Autodesk Fusion 360 part; units mm, degrees
(part 5 of 5)
  constraint perpendicular L8 L9
  constraint parallel L8 L10
  constraint parallel L9 L11
  constraint coincident P0 L0.end
  constraint coincident P1 L1.end
  constraint coincident P3 L0.start
  constraint coincident P9 L15.start
  constraint coincident P10 L15.end
  constraint coincident P11 L16.end
  constraint coincident P8 L17.start
  constraint coincident P15 L18.start
  constraint coincident P12 L19.start
  constraint coincident P13 L20.start
  constraint coincident P14 L20.end
  constraint midpoint L12 A0.centre
  constraint midpoint L13 A1.centre
  constraint midpoint L14 A2.centre
  constraint coincident P2 L2.end
  constraint midpoint L23 A3.centre
  constraint equal A0 A1
  constraint equal A1 A3
  constraint equal A2 A3
  constraint horizontal L64
  constraint perpendicular L57 L64
  constraint parallel L57 L62
  constraint coincident P28 P16
  constraint coincident P17 L55.start
  constraint coincident P18 L54.start
  constraint coincident P24 L59.end
  constraint coincident P29 L58.end
  constraint coincident P20 L70.start
  constraint coincident P30 L63.end
  constraint coincident P22 L56.end
  constraint coincident P33 L56.start
  constraint coincident P31 L58.start
  constraint coincident P32 L65.start
  constraint coincident P23 L65.end
  constraint midpoint A7.centre L73
  constraint midpoint A4.centre L54
  constraint midpoint A6.centre L68
  constraint coincident P19 L59.start
  constraint midpoint A5.centre L67
  constraint equal A4 A7
  constraint equal A4 A5
  constraint equal A5 A6
  constraint horizontal L123
  constraint perpendicular L123 L131
  constraint parallel L130 L131
  constraint coincident P46 P40
  constraint coincident P39 L126.start
  constraint coincident P38 L120.start
  constraint coincident P37 L118.end
  constraint coincident P47 L119.start
  constraint coincident P42 L119.end
  constraint coincident P48 L128.end
  constraint coincident P35 L117.end
  constraint coincident P44 L117.start
  constraint coincident P52 L129.start
  constraint coincident P50 L133.start
  constraint coincident P36 L125.start
  constraint midpoint A11.centre L132
  constraint midpoint A10.centre L122
  constraint midpoint A9.centre L121
  constraint coincident P41 L118.start
  constraint midpoint A8.centre L127
  constraint equal A10 A11
  constraint equal A8 A10
  constraint equal A8 A9
  measures "d633" distance of P2 L11
  measures "d634" distance of P3 L9
  measures "d635" distance of P0 L10
  measures "d636" distance of P3 L8
  measures "d637" diameter of A0
  measures "d664" distance of P19 L62
  measures "d665" distance of P24 L57
  measures "d666" distance of P17 L69
  measures "d667" distance of P24 L64
  measures "d668" diameter of A7
  measures "d670" distance of P41 L130
  measures "d671" distance of P37 L131
  measures "d672" distance of P39 L124
  measures "d673" distance of P37 L123
  measures "d674" diameter of A11
extrude "Extrude4''''" add sketch "Sketch2 (5)" along normal blind 3.6 separate body contours L0 L3 L22 | L0 L1 L15 | L2 L3 L21 | L1 L2 L17 | L8 L9 L10 L11 | L24 S0 S1 S2 S3 S4 S5 S6 L25 S7 S8 S9 S10 S11 S12 S13 L26 S14 S15 S16 S17 S18 S19 S20 S21 S22 S23 S24 S25 S26 | L27 L28 L29 L30 | L31 S27 S28 S29 S30 S31 S32 S33 S34 S35 S36 S37 S38 S39 S40 S41 S42 S43 S44 | S45 S46 S47 S48 S49 S50 S51 S52 S53 | L32 L33 L34 S54 S55 S56 S57 S58 S59 S60 L35 L36 L37 S61 S62 S63 S64 S65 L38 L39 L40 S66 S67 S68 S69 S70 L41 L42 | L43 L44 L45 S71 S72 S73 S74 S75 S76 S77 L46 L47 L48 S78 S79 S80 S81 S82 L49 L50 L51 S83 S84 S85 S86 S87 L52 L53 picked at (11.9917, 14.9333) picked at (11.9917, -11.1667) picked at (-11.9917, 14.9333) picked at (-11.9917, -11.1667) picked at (16.2215, -1.3333) picked at (4.9489, -15.6243) picked at (3.366, -14.1398) picked at (2.568, -15.6926) picked at (1.6677, -15.419) picked at (0.132, -15.1003) picked at (-3.3591, -15.1003) makes body 21 in component "display trial"
extrude "Extrude5''''" cut sketch "Sketch1 (7)" along normal blind 2.5 from surface at -4 contours A0 | A1 | A2 | A3 picked at (-16.5962, -15.4559) picked at (16.6171, -15.5472) picked at (16.0634, 19.1784) picked at (-16.4833, 19.2742) bodies 20 in component "display trial"
extrude "Extrude53" cut sketch "Display cutout (2)" against normal blind 2.5 contours A0 | A1 | A2 | A3 picked at (-46.5866, -131.8202) picked at (-13.9366, -131.8202) picked at (-46.0119, -97.0946) picked at (-13.6923, -97.7089) bodies 5 in component "GM67 + printer"
extrude "Extrude54" cut sketch "SCanner support" against normal up to surface (4 mm away) contours A8 | A9 picked at (14.888, -97.705) picked at (48.012, -96.756) bodies 5 in component "GM67 + printer"
extrude "Extrude55" add sketch "Display cutout (2)" along normal up to surface (1.5 mm away) from surface at -4 contours L14 L22 L23 L24 L25 L33 | L15 L22 L23 L24 L25 L34 picked at (-16.675, -118.5474) picked at (-42.825, -118.5474) bodies 5 in component "GM67 + printer"
extrude "Extrude6'''" add sketch "Sketch2 (5)" along normal blind 3.4 separate body contours L55 L61 L71 | L55 L60 L63 | L59 L61 L66 | L59 L60 L72 | L57 L62 L64 L69 | L74 S88 S89 S90 S91 S92 S93 S94 L75 S95 S96 S97 S98 S99 S100 S101 L76 S102 S103 S104 S105 S106 S107 S108 S109 S110 S111 S112 S113 S114 | L77 L78 L79 L80 | L81 L82 L83 L84 L85 L86 L87 L88 L89 L90 L91 | L92 L93 L94 | L95 L96 L97 S115 S116 S117 S118 S119 S120 S121 L98 L99 L100 S122 S123 S124 S125 S126 L101 L102 L103 S127 S128 S129 S130 S131 L104 L105 | L106 L107 L108 S132 S133 S134 S135 S136 S137 S138 L109 L110 L111 S139 S140 S141 S142 S143 L112 L113 L114 S144 S145 S146 S147 S148 L115 L116 picked at (-59.0083, -11.1667) picked at (-82.9917, -11.1667) picked at (-59.0083, 14.9333) picked at (-82.9917, 14.9333) picked at (-54.7785, -1.3333) picked at (-66.0511, -15.6243) picked at (-67.634, -14.1398) picked at (-69.7384, -16.1548) picked at (-69.1797, -15.5068) picked at (-70.868, -15.1003) picked at (-74.3591, -15.1003) makes body 22 in component "display trial"
extrude "Extrude7''" add sketch "Sketch2 (5)" along normal blind 3.2 separate body contours L118 L120 L125 | L120 L126 L134 | L118 L135 L136 | L119 L126 L136 | L123 L124 L130 L131 | L137 S149 S150 S151 S152 S153 S154 S155 L138 S156 S157 S158 S159 S160 S161 S162 L139 S163 S164 S165 S166 S167 S168 S169 S170 S171 S172 S173 S174 S175 | L140 L141 L142 L143 | L144 L145 S176 S177 S178 S179 S180 S181 S182 S183 S184 L146 S185 S186 S187 S188 S189 S190 S191 S192 S193 L147 | L148 L149 L150 S194 S195 S196 S197 S198 S199 S200 L151 L152 L153 S201 S202 S203 S204 S205 L154 L155 L156 S206 S207 S208 S209 S210 L157 L158 | L159 L160 L161 S211 S212 S213 S214 S215 S216 S217 L162 L163 L164 S218 S219 S220 S221 S222 L165 L166 L167 S223 S224 S225 S226 S227 L168 L169 picked at (-137.9917, 14.9333) picked at (-137.9917, -11.1667) picked at (-114.0083, 14.9333) picked at (-114.0083, -11.1667) picked at (-109.7785, -1.3333) picked at (-121.0511, -15.6243) picked at (-122.634, -14.1398) picked at (-124.0965, -14.118) picked at (-125.868, -15.1003) picked at (-129.3591, -15.1003) makes body 23 in component "display trial"
extrude "Extrude8'''" cut sketch "Sketch2 (5)" against normal blind 1.5 from surface at 3.6 contours L24 S0 S1 S2 S3 S4 S5 S6 L25 S8 S9 S10 S11 S12 S13 L26 S14 S15 S16 S17 S18 S19 S20 S21 S22 S23 S24 S25 S26 | L27 L28 L29 L30 | L31 S27 S28 S29 S30 S31 S32 S33 S34 S35 S36 S37 S38 S39 S40 S41 S42 S43 S44 | L32 L33 L34 S54 S55 S56 S57 S58 S59 S60 L35 L36 L37 S61 S62 S63 S64 S65 L38 L39 L40 S66 S67 S68 S69 S70 L41 L42 | L43 L44 L45 S71 S72 S73 S74 S75 S76 S77 L46 L47 L48 S78 S79 S80 S81 S82 L49 L50 L51 S83 S84 S85 S86 S87 L52 L53 picked at (4.9451, -15.6266) picked at (3.366, -14.1398) picked at (2.568, -15.6926) picked at (0.132, -15.1003) picked at (-3.3591, -15.1003) bodies 21 in component "display trial"
extrude "Extrude9" cut sketch "Sketch2 (5)" against normal blind 1.5 from surface at 3.4 contours L74 S88 S89 S90 S91 S92 S93 S94 L75 S96 S97 S98 S99 S100 S101 L76 S102 S103 S104 S105 S106 S107 S108 S109 S110 S111 S112 S113 S114 | L77 L78 L79 L80 | L81 L82 L83 L84 L85 L86 L87 L88 L89 L90 L91 | L95 L96 L97 S115 S116 S117 S118 S119 S120 S121 L98 L99 L100 S122 S123 S124 S125 S126 L101 L102 L103 S127 S128 S129 S130 S131 L104 L105 | L106 L107 L108 S132 S133 S134 S135 S136 S137 S138 L109 L110 L111 S139 S140 S141 S142 S143 L112 L113 L114 S144 S145 S146 S147 S148 L115 L116 picked at (-66.0549, -15.6266) picked at (-67.634, -14.1398) picked at (-69.7384, -16.1548) picked at (-70.868, -15.1003) picked at (-74.3591, -15.1003) bodies 22 in component "display trial"
extrude "Extrude10" cut sketch "Sketch2 (5)" against normal blind 1.5 from surface at 3.2 contours L137 S149 S150 S151 S152 S153 S154 S155 L138 S157 S158 S159 S160 S161 S162 L139 S163 S164 S165 S166 S167 S168 S169 S170 S171 S172 S173 S174 S175 | L140 L141 L142 L143 | L144 L145 S176 S177 S178 S179 S180 S181 S182 S183 S184 L146 S185 S186 S187 S188 S189 S190 S191 S192 S193 L147 | L148 L149 L150 S194 S195 S196 S197 S198 S199 S200 L151 L152 L153 S201 S202 S203 S204 S205 L154 L155 L156 S206 S207 S208 S209 S210 L157 L158 | L159 L160 L161 S211 S212 S213 S214 S215 S216 S217 L162 L163 L164 S218 S219 S220 S221 S222 L165 L166 L167 S223 S224 S225 S226 S227 L168 L169 picked at (-121.0549, -15.6266) picked at (-122.634, -14.1398) picked at (-124.0965, -14.118) picked at (-125.868, -15.1003) picked at (-129.3591, -15.1003) bodies 23 in component "display trial"
sketch "Sketch1 (8)" plane through (0, 0, 0) normal (0, 1, 0) x (1, 0, 0) in component "Bottom LID - Printer"
  line L0 (0, -115) -> (4, -115)
  arc A0 (19, -100) -> (4, -115) centre (19, -115) ccw
  line L1 (19, -100) -> (43.5, -100)
  arc A1 (43.5, -100) -> (53.5, -90) centre (43.5, -90) ccw
  line L2 (53.5, -90) -> (53.5, -10)
  arc A2 (53.5, -10) -> (43.5, 0) centre (43.5, -10) ccw
  line L3 (43.5, 0) -> (0, 0)
  line L4 (0, 0) -> (0, -115)
  line L5 (49.5, -10) -> (49.5, -90)
  arc A3 (43.5, -96) -> (49.5, -90) centre (43.5, -90) ccw
  line L6 (43.5, -96) -> (4, -96)
  line L7 (4, -96) -> (4, -4)
  line L8 (4, -4) -> (43.5, -4)
  arc A4 (49.5, -10) -> (43.5, -4) centre (43.5, -10) ccw
  line L9 (12, -4) -> (4, -4)
  line L10 (4, -4) -> (4, -12)
  arc A5 (4, -12) -> (12, -4) centre (4, -4) ccw
  line L11 (4, -88) -> (4, -96)
  line L12 (4, -96) -> (12, -96)
  arc A6 (12, -96) -> (4, -88) centre (4, -96) ccw
  arc A7 (45.5, -10) -> (43.5, -8) centre (43.5, -10) ccw
  arc A8 (43.5, -92) -> (45.5, -90) centre (43.5, -90) ccw
  line L13 (45.5, -10) -> (45.5, -90)
  arc A9 (8, -15.3137) -> (15.3137, -8) centre (4, -4) ccw
  arc A10 (15.3137, -92) -> (8, -84.6863) centre (4, -96) ccw
  line L14 (15.3137, -8) -> (43.5, -8)
  line L15 (8, -84.6863) -> (8, -15.3137)
  line L16 (43.5, -92) -> (15.3137, -92)
  circle A11 centre (6.8284, -6.8284) radius 1.75
  circle A12 centre (6.8284, -6.8284) radius 2.8
  circle A13 centre (6.8284, -93.1716) radius 1.75
  circle A14 centre (6.8284, -93.1716) radius 2.8
  line L17 (15.3137, -92) -> (15.3137, -96)
  line L18 (15.3137, -8) -> (15.3137, -4)
  line L19 (40.3137, -96) -> (40.3137, -92)
  line L20 (40.3137, -8) -> (40.3137, -4)
  point P0 (6.8284, -6.8284)
  point P1 (6.8284, -93.1716)
  dimension "d698" = 3.5
  dimension "d699" = 5.6
  dimension "d707" = 25
  constraint concentric A5 A9
  constraint concentric A4 A7
  constraint concentric A3 A8
  constraint tangent A8 L16
  constraint tangent A7 L13
  constraint tangent A8 L13
  constraint coincident P0 A11.centre
  constraint concentric A11 A12
  constraint coincident P1 A13.centre
  constraint equal A12 A14
  constraint equal A11 A13
  constraint coincident L6 L17.end
  constraint perpendicular L6 L17
  constraint coincident L8 L18.end
  constraint perpendicular L8 L18
  constraint coincident L6 L19.start
  constraint coincident L16 L19.end
  constraint perpendicular L16 L19
  constraint coincident L14 L20.start
  constraint coincident L8 L20.end
  constraint perpendicular L8 L20
  constraint collinear L19 L20
  measures "d698" diameter of A11
  measures "d699" diameter of A12
  measures "d707" distance of L17 L19.end
extrude "Extrude1''''''''''" add sketch "Sketch1 (8)" against normal blind 8 separate body contours L5 A3 L6 L8 A4 A7 A8 L13 L14 L16 L19 L20 | L8 L14 L18 L20 | L6 L16 L17 L19 | L6 L7 L8 A5 A6 A9 A10 L15 L17 L18 picked at (48.1667, -63.3333) picked at (31.9804, -6.6667) picked at (31.9804, -94.6667) picked at (5.3333, -61.5621) makes body 24 in component "Bottom LID - Printer"
extrude "Extrude3'''''''" add sketch "Sketch1 (8)" along normal blind 4 contours L0 A0 L1 A1 L2 A2 L3 L4 | L5 A3 L6 L8 A4 A7 A8 L13 L14 L16 L19 L20 | L8 L14 L18 L20 | L6 L16 L17 L19 | L6 L7 L8 A5 A6 A9 A10 L15 L17 L18 | A7 A8 L13 A9 A10 L14 L15 L16 | L7 L8 L9 L10 A5 | L6 L7 L11 L12 A6 | A12 | A14 picked at (8.9635, -98.1271) picked at (48.1667, -63.3333) picked at (31.9804, -6.6667) picked at (31.9804, -94.6667) picked at (5.3333, -61.5621) picked at (33.5434, -61.8009) picked at (11.0202, -4.7965) picked at (11.0202, -95.2035) picked at (9.268, -6.9675) picked at (9.268, -93.3107) bodies 24 in component "Bottom LID - Printer"
extrude "Extrude5'''''" add sketch "Sketch1 (8)" against normal blind 2.5 contours L7 L8 L9 L10 A5 | L6 L7 L11 L12 A6 | A12 | A14 picked at (11.0202, -4.7965) picked at (11.0202, -95.2035) picked at (9.268, -6.9675) picked at (9.268, -93.3107) bodies 24 in component "Bottom LID - Printer"
extrude "Extrude6''''" cut sketch "Sketch1 (8)" against normal blind 3 from surface at 4 contours A12 | A14 picked at (9.268, -6.9675) picked at (9.268, -93.3107) bodies 24 in component "Bottom LID - Printer"
extrude "Extrude7'''" add sketch "Sketch1 (8)" against normal blind 5 from surface at -8 contours L8 L14 L18 L20 | L6 L16 L17 L19 picked at (31.9804, -6.6667) picked at (31.9804, -94.6667) bodies 24 in component "Bottom LID - Printer"
fillet "Fillet2'" radius 2 8 edges at (15.3137, -8, 6) (15.3137, -13, 6) (40.3137, -13, 6) (40.3137, -8, 6) (40.3137, -8, 94) (40.3137, -13, 94) (15.3137, -13, 94) (15.3137, -8, 94) on bodies 24 in component "Bottom LID - Printer"
sketch "Sketch1 (9)" plane through (0, 0, 0) normal (0, 1, 0) x (1, 0, 0) in component "Top lid"
  line L0 (0, 0) -> (183.0748, 0)
  line L1 (53.5, -96) -> (53.5, -4)
  line L2 (196.0652, -7.5) -> (240.6025, -84.641)
  line L3 (192.6011, -9.5) -> (237.1384, -86.641)
  line L4 (4, -4) -> (183.0748, -4)
  arc A0 (109.3397, -4) -> (125.3397, -4) centre (117.3397, -4) ccw
  arc A1 (53.5, -12) -> (61.5, -4) centre (53.5, -4) ccw
  arc A2 (61.5, -96) -> (53.5, -88) centre (53.5, -96) ccw
  line L5 (125.3397, -96) -> (19, -96)
  line L6 (125.3397, -100) -> (19, -100)
  arc A3 (141.7942, -105.5) -> (125.3397, -96) centre (125.3397, -115) ccw
  arc A4 (138.3301, -107.5) -> (125.3397, -100) centre (125.3397, -115) ccw
  line L7 (154, -134.641) -> (138.3301, -107.5)
  line L8 (157.4641, -132.641) -> (141.7942, -105.5)
  line L9 (179.9994, -4) -> (179.9994, -6.8969)
  line L10 (181.9766, -9.7171) -> (186.9578, -11.5237)
  arc A5 (179.9994, -6.8969) -> (181.9766, -9.7171) centre (182.9994, -6.8969) ccw
  line L11 (192.6011, -9.5) -> (189.4806, -11.3016)
  arc A6 (196.0652, -7.5) -> (183.0748, 0) centre (183.0748, -15) ccw
  arc A7 (186.9578, -11.5237) -> (189.4806, -11.3016) centre (187.9806, -8.7035) ccw
  arc A8 (154, -134.641) -> (174.4904, -140.1314) centre (166.9904, -127.141) ccw
  arc A9 (157.4641, -132.641) -> (172.4904, -136.6673) centre (166.9904, -127.141) ccw
  spline S0 degree 2 poles (157.4641, -132.641) (166.9904, -127.141) (172.4904, -136.6673) knots 0 0 0 1.944544 1.944544 1.944544 weights 1 3 1
  line L12 (233.1122, -101.6673) -> (172.4904, -136.6673)
  line L13 (235.1122, -105.1314) -> (174.4904, -140.1314)
  arc A10 (233.1122, -101.6673) -> (237.1384, -86.641) centre (227.6122, -92.141) ccw
  spline S1 degree 2 poles (233.1122, -101.6673) (227.6122, -92.141) (237.1384, -86.641) knots 0 0 0 1.944544 1.944544 1.944544 weights 1 3 1
  arc A11 (235.1122, -105.1314) -> (240.6025, -84.641) centre (227.6122, -92.141) ccw
  line L14 (53.5, -4) -> (53.5, 0)
  line L15 (53.5, -96) -> (53.5, -100)
  circle A12 centre (56.3284, -93.1716) radius 1.75
  circle A13 centre (165.1786, -133.9025) radius 1.75
  circle A14 centre (234.3736, -93.9527) radius 1.75
  arc A15 (125.3397, -96) -> (109.3397, -96) centre (117.3397, -96) ccw
  circle A16 centre (117.3397, -93.1716) radius 1.75
  circle A17 centre (56.3284, -6.8284) radius 1.75
  circle A18 centre (117.3397, -6.8284) radius 1.75
  circle A19 centre (185.872, -7.6542) radius 1.75
  circle A20 centre (56.3284, -6.8284) radius 2.75
  circle A21 centre (117.3397, -6.8284) radius 2.75
  circle A22 centre (185.872, -7.6542) radius 2.75
  circle A23 centre (117.3397, -93.1716) radius 2.75
  circle A24 centre (56.3284, -93.1716) radius 2.75
  circle A25 centre (234.3736, -93.9527) radius 2.75
  circle A26 centre (165.1786, -133.9025) radius 2.75
  arc A27 (43.5, -100) -> (53.5, -90) centre (43.5, -90) ccw
  line L16 (43.5, -100) -> (125.3397, -100)
  arc A28 (53.5, -10) -> (43.5, 0) centre (43.5, -10) ccw
  line L17 (183.0748, 0) -> (43.5, 0)
  arc A29 (192.6011, -9.5) -> (183.0748, -4) centre (183.0748, -15) ccw
  line L18 (158.9576, -127.2278) -> (145.2583, -103.5)
  arc A30 (145.2583, -103.5) -> (128.7396, -92.2527) centre (125.3397, -115) ccw
  arc A31 (64.8137, -92) -> (57.5, -84.6863) centre (53.5, -96) ccw
  arc A32 (57.5, -15.3137) -> (64.8137, -8) centre (53.5, -4) ccw
  arc A33 (106.026, -8) -> (128.6534, -8) centre (117.3397, -4) ccw
  arc A34 (176.0869, -8) -> (180.6127, -13.4774) centre (182.9994, -6.8969) ccw
  line L19 (180.6127, -13.4774) -> (185.5939, -15.284)
  arc A35 (185.5939, -15.284) -> (191.4806, -14.7657) centre (187.9806, -8.7035) ccw
  line L20 (191.1313, -14.9543) -> (231.7036, -85.2276)
  line L21 (227.6989, -100.1738) -> (173.9038, -131.2325)
  spline S2 degree 3 poles (227.6989, -100.1738) (227.0051, -98.8648) (226.5887, -97.9787) (226.2602, -97.1692) (225.8173, -96.0779) (225.5432, -95.1491) (225.4386, -94.1266) (225.3307, -93.0717) (225.4574, -91.9156) (225.8682, -90.8802) (226.2709, -89.8653) (226.8901, -89.0216) (227.6185, -88.2841) (228.2608, -87.6338) (228.9814, -87.0511) (230.0273, -86.3265) (230.495, -86.0025) (231.0263, -85.6518) (231.7036, -85.2276) knots 0.158277 0.158277 0.158277 0.158277 0.396251 0.396251 0.396251 0.717027 0.717027 0.717027 1.047986 1.047986 1.047986 1.372407 1.372407 1.372407 1.658475 1.658475 1.658475 1.786413 1.786413 1.786413 1.786413
  spline S3 degree 3 poles (158.9576, -127.2278) (160.2666, -126.534) (161.1527, -126.1176) (161.9622, -125.789) (163.0535, -125.3462) (163.9823, -125.0721) (165.0048, -124.9675) (166.0597, -124.8596) (167.2158, -124.9862) (168.2512, -125.3971) (169.2661, -125.7998) (170.1098, -126.4189) (170.8473, -127.1473) (171.4976, -127.7896) (172.0803, -128.5103) (172.8049, -129.5561) (173.1289, -130.0238) (173.4796, -130.5551) (173.9038, -131.2325) knots 0.158277 0.158277 0.158277 0.158277 0.396251 0.396251 0.396251 0.717027 0.717027 0.717027 1.047986 1.047986 1.047986 1.372407 1.372407 1.372407 1.658475 1.658475 1.658475 1.786412 1.786412 1.786412 1.786412
  arc A36 (128.7396, -92.2527) -> (106.026, -92) centre (117.3397, -96) ccw
  line L22 (106.026, -92) -> (64.8137, -92)
  line L23 (57.6284, -92) -> (57.5, -92)
  line L24 (57.5, -92) -> (57.5, -91.8716)
  line L25 (4, -8) -> (53.298, -8)
  line L26 (57.5, -84.6863) -> (57.5, -15.3137)
  line L27 (64.8137, -8) -> (106.026, -8)
  line L28 (128.6534, -8) -> (176.0869, -8)
  arc A37 (189.1369, -11.5) -> (189.1237, -11.4772) centre (183.0748, -15) ccw
  arc A38 (183.1439, -8.0003) -> (183.0748, -8) centre (183.0748, -15) ccw
  point P0 (56.3284, -6.8284)
  point P1 (56.3284, -93.1716)
  point P2 (117.3397, -93.1716)
  point P3 (117.3397, -6.8284)
  point P4 (185.872, -7.6542)
  point P5 (234.3736, -93.9527)
  point P6 (165.1786, -133.9025)
  point P7 (141.7942, -105.5)
  dimension "d715" = 3.5
  dimension "d716" = 5.5
  dimension "d729" = 4
  dimension "d730" = 4
  constraint coincident L1.end A1.centre
  constraint coincident L0 L14.end
  constraint perpendicular L0 L14
  constraint coincident L1.start A2.centre
  constraint coincident L6 L15.end
  constraint perpendicular L6 L15
  constraint coincident P1 A12.centre
  constraint coincident P6 A13.centre
  constraint coincident P5 A14.centre
  constraint coincident P2 A16.centre
  constraint coincident P0 A17.centre
  constraint coincident P3 A18.centre
  constraint coincident P4 A19.centre
  constraint equal A18 A19
  constraint equal A12 A19
  constraint equal A12 A16
  constraint equal A13 A16
  constraint equal A13 A14
  constraint equal A14 A17
  constraint concentric A17 A20
  constraint concentric A18 A21
  constraint concentric A12 A24
  constraint equal A20 A21
  constraint equal A21 A22
  constraint equal A22 A24
  constraint equal A23 A24
  constraint equal A23 A26
  constraint equal A25 A26
  constraint concentric A3 A30
  constraint concentric A15 A36
  constraint collinear L22 L23
  constraint concentric A2 A31
  constraint coincident A12 L23.start
  constraint coincident A12 L24.end
  constraint concentric A29 A37
  constraint collinear L25 L27
  constraint coincident A28 L25.end
  constraint concentric A1 A32
  constraint concentric A0 A33
  constraint concentric A5 A34
  constraint coincident A22 A38.start
  constraint concentric A37 A38
  constraint coincident A7 A37.end
  constraint coincident A35 L20.start
  measures "d715" diameter of A17
  measures "d716" diameter of A20
extrude "Extrude1'''''''''''" add sketch "Sketch1 (9)" along normal blind 4 separate body contours L0 L4 L14 A28 L17 | L0 L2 L3 L4 L5 L6 A3 A4 L7 L8 A6 A8 A9 L12 L13 A10 A11 L14 L15 L16 L17 A29 | L1 L4 A28 | L1 L4 A1 | L1 L3 L4 A0 A1 A2 L5 A3 L8 L9 L10 A5 L11 A7 S0 L12 S1 A15 | L4 A0 | L1 A2 L5 | L1 L5 A27 | L4 L9 L10 A5 L11 A7 A29 | L5 L6 L15 A27 L16 | L5 A15 | A10 S1 | A9 S0 | A20 | A21 | A22 | A23 | A24 | A25 | A26 | L18 A30 A31 A32 A33 A34 L19 A35 L20 L21 S2 S3 A36 L22 L26 L27 L28 picked at (52.5458, -2.332) picked at (115.3048, -1.3333) picked at (52.4315, -4.4133) picked at (54.4874, -10.4356) picked at (206.9569, -37.0318) picked at (111.2103, -4.9425) picked at (54.4874, -89.5644) picked at (52.4013, -95.6412) picked at (189.8421, -9.4152) picked at (52.5458, -97.668) picked at (111.2103, -95.0575) picked at (235.3087, -89.4652) picked at (169.6485, -134.9038) picked at (58.7283, -7.052) picked at (119.7462, -6.965) picked at (183.4629, -7.7491) picked at (115.0805, -94.0114) picked at (55.969, -90.787) picked at (233.9714, -96.3292) picked at (164.8626, -136.292) picked at (185.7087, -68.7412) makes body 25 in component "Top lid"
extrude "Extrude2'''''''" cut sketch "Sketch1 (9)" against normal blind 3 from surface at 4 contours A20 | A21 | A22 | A23 | A24 | A25 | A26 picked at (58.7283, -7.052) picked at (119.7462, -6.965) picked at (183.4629, -7.7491) picked at (115.0805, -94.0114) picked at (55.969, -90.787) picked at (233.9714, -96.3292) picked at (164.8626, -136.292) bodies 25 in component "Top lid"
extrude "Extrude3''''''''" add sketch "Sketch1 (9)" against normal blind 2.5 contours L1 L3 L4 A0 A1 A2 L5 A3 L8 L9 L10 A5 L11 A7 S0 L12 S1 A15 picked at (206.9569, -37.0318) bodies 25 in component "Top lid"
extrude "Extrude4'''''" add sketch "Sketch1 (9)" against normal blind 2.5 contours L1 L4 A1 | L4 A0 | L1 A2 L5 | L4 L9 L10 A5 L11 A7 A29 | L5 A15 | A10 S1 | A9 S0 | A20 | A21 | A22 | A23 | A24 | A25 | A26 picked at (54.4874, -10.4356) picked at (111.2103, -4.9425) picked at (54.4874, -89.5644) picked at (189.8421, -9.4152) picked at (111.2103, -95.0575) picked at (235.3087, -89.4652) picked at (169.6485, -134.9038) picked at (58.7283, -7.052) picked at (119.7462, -6.965) picked at (183.4629, -7.7491) picked at (115.0805, -94.0114) picked at (55.969, -90.787) picked at (233.9714, -96.3292) picked at (164.8626, -136.292) bodies 25 in component "Top lid"
sketch "Sketch1 (10)" plane through (0, 0, 0) normal (0, 1, 0) x (1, 0, 0) in component "Scanner GM67"
  line L0 (0, 0) -> (165.7543, 0)
  line L1 (178.7446, -7.5) -> (207.1218, -56.6506)
  line L2 (201.6314, -77.141) -> (166.9904, -97.141)
  line L3 (146.5, -91.6506) -> (138.3301, -77.5)
  line L4 (125.3397, -70) -> (19, -70)
  line L5 (4, -85) -> (4, -112)
  line L6 (1, -115) -> (0, -115)
  line L7 (0, -115) -> (0, 0)
  arc A0 (178.7446, -7.5) -> (165.7543, 0) centre (165.7543, -15) ccw
  arc A1 (201.6314, -77.141) -> (207.1218, -56.6506) centre (194.1314, -64.1506) ccw
  arc A2 (146.5, -91.6506) -> (166.9904, -97.141) centre (159.4904, -84.1506) ccw
  arc A3 (138.3301, -77.5) -> (125.3397, -70) centre (125.3397, -85) ccw
  arc A4 (19, -70) -> (4, -85) centre (19, -85) ccw
  line L8 (4, -4) -> (165.7543, -4)
  arc A5 (175.2805, -9.5) -> (165.7543, -4) centre (165.7543, -15) ccw
  line L9 (175.2805, -9.5) -> (203.6577, -58.6506)
  arc A6 (199.6314, -73.6769) -> (203.6577, -58.6506) centre (194.1314, -64.1506) ccw
  line L10 (199.6314, -73.6769) -> (164.9904, -93.6769)
  arc A7 (149.9641, -89.6506) -> (164.9904, -93.6769) centre (159.4904, -84.1506) ccw
  line L11 (149.9641, -89.6506) -> (141.7942, -75.5)
  arc A8 (141.7942, -75.5) -> (125.3397, -66) centre (125.3397, -85) ccw
  line L12 (125.3397, -66) -> (19, -66)
  arc A9 (19, -66) -> (4, -73.3381) centre (19, -85) ccw
  line L13 (4, -73.3381) -> (4, -4)
  arc A10 (1, -115) -> (4, -112) centre (1, -112) ccw
  arc A11 (4, -14) -> (14, -4) centre (4, -4) ccw
  line L14 (4, -4) -> (11.0711, -11.0711) construction
  circle A12 centre (7.5355, -7.5355) radius 2
  line L15 (19, -85) -> (19, -51) construction
  arc A13 (4, -51) -> (19, -66) centre (19, -51) ccw
  line L16 (19, -66) -> (4, -66) construction
  circle A14 centre (7, -66) radius 2
  line L17 (159.4904, -84.1506) -> (154, -104.641) construction
  spline S0 degree 2 poles (149.9641, -89.6506) (159.4904, -84.1506) (164.9904, -93.6769) knots 0 0 0 1.944544 1.944544 1.944544 weights 1 3 1
  circle A15 centre (157.6786, -90.9121) radius 2
  line L18 (175.2805, -9.5) -> (172.1601, -11.3016)
  line L19 (162.6789, -4) -> (162.6789, -6.8969)
  line L20 (164.656, -9.7171) -> (169.6373, -11.5237)
  arc A16 (162.6789, -6.8969) -> (164.656, -9.7171) centre (165.6789, -6.8969) ccw
  arc A17 (169.6373, -11.5237) -> (172.1601, -11.3016) centre (170.6601, -8.7035) ccw
  spline S1 degree 2 poles (199.6314, -73.6769) (194.1314, -64.1506) (203.6577, -58.6506) knots 0 0 0 1.944543 1.944543 1.944543 weights 1 3 1
  line L21 (194.1314, -64.1506) -> (214.6218, -69.641) construction
  circle A18 centre (200.8929, -65.9624) radius 2
  line L22 (162.6789, -4) -> (175.2805, -9.5) construction
  arc A19 (125.3397, -66) -> (109.3397, -66) centre (117.3397, -66) ccw
  line L23 (117.3397, -66) -> (117.3397, -58) construction
  circle A20 centre (117.3397, -62) radius 2
  line L24 (4, -85) -> (0, -85)
  line L25 (168.9797, -6.75) -> (167.1467, -10.6204) construction
  circle A21 centre (168.5515, -7.6542) radius 2
  circle A22 centre (7.5355, -7.5355) radius 2.25
  circle A23 centre (168.5515, -7.6542) radius 2.25
  circle A24 centre (200.8929, -65.9624) radius 2.25
  circle A25 centre (117.3397, -62) radius 2.25
  circle A26 centre (7, -66) radius 2.25
  circle A27 centre (157.6786, -90.9121) radius 2.25
  line L26 (4, -38.669) -> (192.1213, -38.669) construction
  line L27 (157, -6.669) -> (87, -6.669)
  line L28 (87, -6.669) -> (87, -56.669)
  line L29 (87, -56.669) -> (157, -56.669)
  line L30 (157, -56.669) -> (157, -6.669)
  line L31 (157, -6.669) -> (87, -56.669) construction
  line L32 (87, -6.669) -> (157, -56.669) construction
  line L33 (155.04, -8.604) -> (88.96, -8.604)
  line L34 (88.96, -8.604) -> (88.96, -54.734) construction
  line L35 (88.96, -54.734) -> (155.04, -54.734) construction
  line L36 (155.04, -54.734) -> (155.04, -8.604) construction
  line L37 (155.04, -8.604) -> (88.96, -54.734) construction
  line L38 (88.96, -8.604) -> (155.04, -54.734) construction
  circle A28 centre (88.96, -54.734) radius 0.95
  circle A29 centre (88.96, -54.734) radius 3.45
  circle A30 centre (155.04, -54.734) radius 0.95
  circle A31 centre (155.04, -54.734) radius 3.45
  circle A32 centre (155.04, -8.604) radius 0.95
  circle A33 centre (155.04, -8.604) radius 3.45
  circle A34 centre (88.96, -8.604) radius 3.45
  circle A35 centre (88.96, -8.604) radius 0.95
  point P0 (214.6218, -69.641)
  point P1 (154, -104.641)
  point P2 (134, -70)
  point P3 (4, -70)
  point P4 (4, -115)
  point P5 (170.9504, -12)
  point P6 (162.6789, -9)
  point P7 (122, -31.669)
  point P8 (122, -31.669)
  point P9 (122, -31.669)
  dimension "d1_1" = 130
  dimension "d2_1" = 70
  dimension "d3_1" = 70
  dimension "d4_1" = 40
  dimension "d5_1" = 4
  dimension "d7_1" = 45
  dimension "d8_1" = 120
  dimension "d9_1" = 4
  dimension "d40_1" = 15
  dimension "d47_1" = 3
  dimension "d84_2" = 10
  dimension "d85_1" = 4
  dimension "d88_1" = 19
  dimension "d94_1" = 15
  dimension "d95_1" = 19
  dimension "d96_1" = 15
  dimension "d97_1" = 15
  dimension "d98_1" = 3
  dimension "d101_1" = 11
  dimension "d102_1" = 15
  dimension "d105_1" = 7
  dimension "d111_1" = 5
  dimension "d112_1" = 5
  dimension "d113_1" = 3
  dimension "d115_1" = 7
  dimension "d120_1" = 8
  dimension "d121_1" = 8
  dimension "d139_1" = 1
  dimension "d147_1" = 0.25
  dimension "d148_1" = 0.25
  dimension "d149_1" = 0.25
  dimension "d150_1" = 0.25
  dimension "d151_1" = 0.25
  dimension "d153_1" = 3.2821
  dimension "d157_1" = 0.25
  dimension "d234_1" = 70
  dimension "d235_1" = 50
  dimension "d236_1" = 66.08
  dimension "d237_1" = 46.13
  dimension "d238_1" = 1.9
  dimension "d239_1" = 2.5
  dimension "d240_1" = 7
  dimension "d241_1" = 118
  constraint coincident L0.start L7.end
  constraint horizontal L0
  constraint perpendicular L1 L2
  constraint parallel L0 L4
  constraint perpendicular L4 L5
  constraint parallel L1 L3
  constraint perpendicular L5 L6
  constraint perpendicular L0 L7
  constraint tangent L0 A0
  constraint tangent L1 A0
  constraint coincident P0 L1
  constraint coincident P0 L2
  constraint tangent L1 A1
  constraint tangent L2 A1
  constraint equal A0 A1
  constraint coincident P1 L2
  constraint coincident P1 L3
  constraint tangent L2 A2
  constraint tangent L3 A2
  constraint equal A0 A2
  constraint coincident P2 L3
  constraint coincident P2 L4
  constraint tangent L3 A3
  constraint tangent L4 A3
  constraint equal A0 A3
  constraint coincident P3 L4
  constraint coincident P3 L5
  constraint tangent L4 A4
  constraint tangent L5 A4
  constraint equal A0 A4
  constraint coincident P4 L5
  constraint coincident P4 L6
  constraint tangent L5 A10
  constraint tangent L6 A10
  constraint coincident L13 A11.start
  constraint coincident L8 A11.end
  constraint coincident L8.start L13.end
  constraint midpoint A11 L14.end
  constraint midpoint L14 A12.centre
  constraint coincident A4.centre A9.centre
  constraint perpendicular L12 L15
  constraint coincident L13 A13.start
  constraint coincident L15.end A13.centre
  constraint coincident L13 L16.end
  constraint tangent A9 L16
  constraint perpendicular L13 L16
  constraint coincident L16 A14.centre
  constraint equal A12 A14
  constraint coincident A2.centre A7.centre
  constraint coincident P1 L17.end
  constraint coincident L17 A15.centre
  constraint equal A12 A15
  constraint perpendicular L9 L18
  constraint coincident L8 L19.start
  constraint perpendicular L8 L19
  constraint coincident P6 L19
  constraint coincident P6 L20
  constraint tangent L19 A16
  constraint tangent L20 A16
  constraint coincident P5 L20
  constraint coincident P5 L18
  constraint tangent L20 A17
  constraint tangent L18 A17
  constraint equal A16 A17
  constraint coincident A1.centre A6.centre
  constraint coincident P0 L21.end
  constraint coincident L21 A18.centre
  constraint equal A12 A18
  constraint coincident L12 A8.end
  constraint coincident L12 A19.centre
  constraint coincident A19.centre L23.start
  constraint perpendicular L12 L23
  constraint midpoint L23 A20.centre
  constraint equal A12 A20
  constraint coincident L7 L24.end
  constraint perpendicular L7 L24
  constraint midpoint L22 L25.start
  constraint midpoint L20 L25.end
  constraint coincident L25 A21.centre
  constraint equal A12 A21
  constraint midpoint L13 L26.start
  constraint coincident L9 L26.end
  constraint perpendicular L13 L26
  constraint horizontal L27
  constraint perpendicular L27 L28
  constraint parallel L27 L29
  constraint parallel L28 L30
  constraint coincident L31 P9
  constraint coincident L32 P9
  constraint coincident P9 P8
  constraint horizontal L33
  constraint perpendicular L33 L34
  constraint parallel L33 L35
  constraint parallel L34 L36
  constraint coincident L37 P9
  constraint coincident L38 P9
  constraint coincident L34.end L35.start
  constraint coincident L35.end L36.start
  constraint coincident L33.start L36.end
  constraint concentric A32 A33
  constraint coincident L33.end L34.start
  constraint concentric A34 A35
  constraint equal A29 A31
  constraint equal A31 A33
  constraint equal A33 A34
  constraint equal A28 A32
  constraint equal A30 A32
  constraint equal A30 A35
  measures "d1_1" distance of P2 P3
  measures "d2_1" distance of L0 L4
  measures "d3_1" distance of P0 P1
  measures "d4_1" distance of P1 P2
  measures "d5_1" distance of P4 L6.end
  measures "d7_1" distance of P3 P4
  measures "d8_1" angle of L3 L4
  measures "d40_1" radius of A0
  measures "d47_1" radius of A10
  measures "d84_2" radius of A11
  measures "d85_1" diameter of A12
  measures "d88_1" radius of A9
  measures "d94_1" distance of L4.end A4.centre
  measures "d95_1" distance of A4.centre L12
  measures "d96_1" distance of L5.start A4.centre
  measures "d97_1" distance of L12.end L15.end
  measures "d98_1" distance of L13 A14.centre
  measures "d101_1" radius of A7
  measures "d102_1" radius of A2
  measures "d105_1" distance of A2.centre A15.centre
  measures "d111_1" distance of L19.start P6
  measures "d112_1" distance of A5.start P5
  measures "d113_1" radius of A16
  measures "d115_1" distance of A1.centre A18.centre
  measures "d120_1" radius of A19
  measures "d121_1" distance of A8.end A19.centre
  measures "d139_1" distance of L22 A21.centre
  measures "d153_1" distance of L25.end A21.centre
  measures "d234_1" distance of L28.end L29.end
  measures "d235_1" distance of L27.end L28.end
  measures "d236_1" distance of L34.end L35.end
  measures "d237_1" distance of L33.end L34.end
  measures "d238_1" diameter of A28
  measures "d240_1" distance of L26 P9
  measures "d241_1" distance of L13 P9
extrude "Extrude1''''''''''''" [suppressed] in component "Scanner GM67"
sketch "Display cutout (3)" plane through (81.8109, 0, 141.7006) normal (-0.5, 0, -0.866025) x (0, -1, 0) in component "Scanner GM67"
  line L0 (0, -136.0474) -> (0, -96.0474)
  line L1 (-60, -96.0474) -> (-60, -136.0474)
  line L2 (0, -116.0474) -> (-60, -116.0474) construction
  line L3 (0, -96.0474) -> (-60, -96.0474)
  line L4 (-60, -136.0474) -> (0, -136.0474)
  line L5 (-38.325, -103.0474) -> (-38.325, -108.5474)
  line L6 (-43.825, -123.5474) -> (-43.825, -132.5474)
  line L7 (-43.825, -103.0474) -> (-16.175, -103.0474)
  line L8 (-43.825, -132.5474) -> (-43.825, -127.8474)
  line L9 (-43.825, -132.5474) -> (-16.175, -132.5474)
  line L10 (-38.325, -132.5474) -> (-43.825, -132.5474)
  line L11 (-43.825, -127.8474) -> (-38.325, -127.8474)
  line L12 (-38.325, -127.8474) -> (-38.325, -132.5474)
  line L13 (-43.825, -108.5474) -> (-43.825, -103.0474)
  line L14 (-43.825, -108.5474) -> (-43.825, -123.5474)
  line L15 (-16.175, -123.5474) -> (-16.175, -108.5474)
  line L16 (-21.675, -132.5474) -> (-21.675, -127.8474)
  line L17 (-43.825, -123.5474) -> (-16.175, -108.5474) construction
  line L18 (-16.175, -103.0474) -> (-16.175, -108.5474)
  line L19 (-16.175, -132.5474) -> (-16.175, -123.5474)
  line L20 (-21.675, -127.8474) -> (-16.175, -127.8474)
  line L21 (-16.175, -127.8474) -> (-16.175, -132.5474)
  line L22 (-16.175, -108.5474) -> (-43.825, -108.5474)
  line L23 (-16.175, -123.5474) -> (-43.825, -123.5474)
  line L24 (-43.825, -123.5474) -> (-16.175, -123.5474)
  line L25 (-16.175, -108.5474) -> (-43.825, -108.5474)
  line L26 (-21.675, -103.0474) -> (-21.675, -108.5474)
  line L27 (-16.175, -123.5474) -> (-43.825, -108.5474) construction
  line L28 (-16.175, -132.5474) -> (-21.675, -132.5474)
  point P0 (-30, -116.0474)
  point P1 (-30, -116.0474)
  point P2 (-30, -116.0474)
  dimension "d64_1" = 27.65
  dimension "d65_1" = 15
  dimension "d66_1" = 5.5
  dimension "d67_1" = 9
  dimension "d68_1" = 5.5
  dimension "d69_1" = 5.5
  dimension "d70_1" = 4.7
  dimension "d225_1" = 29.5
  dimension "d226_1" = 24.8
  constraint midpoint L0 L2.start
  constraint midpoint L1 L2.end
  constraint horizontal L24
  constraint perpendicular L15 L24
  constraint parallel L24 L25
  constraint parallel L14 L15
  constraint coincident P2 L17
  constraint coincident P2 L27
  constraint perpendicular L13 L22
  constraint parallel L7 L22
  constraint parallel L13 L18
  constraint perpendicular L6 L23
  constraint parallel L9 L23
  constraint parallel L6 L19
  constraint coincident L26.start L7
  constraint coincident L26.end L25
  constraint perpendicular L25 L26
  constraint coincident L5.start L7
  constraint coincident L5.end L22
  constraint perpendicular L5 L22
  constraint horizontal L28
  constraint vertical L16
  constraint horizontal L20
  constraint vertical L21
  constraint collinear L16 L26
  constraint horizontal L10
  constraint vertical L8
  constraint horizontal L11
  constraint vertical L12
  constraint coincident L8.end L6
  constraint coincident L10.start L9
  constraint collinear L5 L12
  constraint collinear L11 L20
  constraint coincident P2 P1
  constraint midpoint L2 P2
  measures "d64_1" distance of L15.end L13.start
  measures "d65_1" distance of L15.end L15.start
  measures "d66_1" distance of L15.end L7.end
  measures "d67_1" distance of L15.start L9.end
  measures "d68_1" distance of L18 L26
  measures "d69_1" distance of L5 L13
  measures "d70_1" distance of L20 L28
  measures "d225_1" distance of L7 L9
  measures "d226_1" distance of L7 L20
extrude "Extrude8''''" [suppressed] in component "Scanner GM67"
sketch "Sensor cutout (3)" plane through (0, 0, 66) normal (0, 0, -1) x (1, 0, 0) in component "Scanner GM67"
  line L0 (125.3397, 0) -> (19, 0)
  line L1 (19, 0) -> (19, -60)
  line L2 (19, -60) -> (125.3397, -60)
  line L3 (125.3397, -60) -> (125.3397, 0)
  line L4 (19, -30) -> (125.3397, -30) construction
  circle A0 centre (69, -30) radius 13
  dimension "d48_1" = 26
  dimension "d49_1" = 50
  constraint midpoint L1 L4.start
  constraint coincident L4 A0.centre
  measures "d48_1" diameter of A0
  measures "d49_1" distance of L4.start A0.centre
extrude "Extrude1'''''''''''''" [suppressed] in component "Scanner GM67"
sketch "Power cutout (3)" plane through (0, 0, 4) normal (0, 0, 1) x (-1, 0, 0) in component "Scanner GM67"
  line L0 (-4, 0) -> (-165.7543, 0)
  line L1 (-165.7543, 0) -> (-165.7543, -60)
  line L2 (-165.7543, -60) -> (-4, -60)
  line L3 (-4, -60) -> (-4, 0)
  line L4 (-4, -30) -> (-165.7543, -30) construction
  circle A0 centre (-34, -30) radius 4
  line L5 (-38.95, -32.8579) -> (-34, -35.7158)
  line L6 (-34, -35.7158) -> (-29.05, -32.8579)
  line L7 (-29.05, -32.8579) -> (-29.05, -27.1421)
  line L8 (-29.05, -27.1421) -> (-34, -24.2842)
  line L9 (-34, -24.2842) -> (-38.95, -27.1421)
  line L10 (-38.95, -27.1421) -> (-38.95, -32.8579)
  line L11 (-102.7993, -29.1827) -> (-102.7993, -29)
  circle A1 centre (-79, -30) radius 4.625
  circle A2 centre (-79, -30) radius 2.25
  circle A3 centre (-79, -30) radius 7.625
  point P0 (-34, -30)
  dimension "d52_1" = 8
  dimension "d53_1" = 30
  dimension "d133_1" = 9.9
  dimension "d191_1" = 3
  dimension "d193_1" = 9.25
  dimension "d194_1" = 4.5
  dimension "d195_1" = 75
  constraint midpoint L3 L4.start
  constraint midpoint L1 L4.end
  constraint coincident L4 P0
  constraint coincident P0 A0.centre
  constraint concentric A1 A2
  constraint coincident L4 A1.centre
  measures "d52_1" diameter of A0
  measures "d53_1" distance of L3 P0
  measures "d133_1" distance of L7 L10
  measures "d193_1" diameter of A1
  measures "d194_1" diameter of A2
  measures "d195_1" distance of L3 A1.centre
extrude "Extrude2''''''''" [suppressed] in component "Scanner GM67"
extrude "Extrude3'''''''''" [suppressed] in component "Scanner GM67"
extrude "Extrude4''''''" [suppressed] in component "Scanner GM67"
extrude "Extrude5''''''" [suppressed] in component "Scanner GM67"
extrude "Extrude7''''" [suppressed] in component "Scanner GM67"
extrude "Extrude8'''''" [suppressed] in component "Scanner GM67"
extrude "Extrude11'" [suppressed] in component "Scanner GM67"
extrude "Extrude12''" [suppressed] in component "Scanner GM67"
extrude "Extrude13'" [suppressed] in component "Scanner GM67"
extrude "Extrude18'" [suppressed] in component "Scanner GM67"
extrude "Extrude19'" [suppressed] in component "Scanner GM67"
sketch "Button cutout (3)" plane through (127.3468, 0, -73.5237) normal (-0.866025, 0, 0.5) x (0, -1, 0) in component "Scanner GM67"
  line L0 (0, 95.8675) -> (0, 152.6218)
  line L1 (0, 152.6218) -> (-57.25, 152.6218)
  line L2 (-57.25, 152.6218) -> (-60, 152.6218)
  line L3 (-60, 152.6218) -> (-60, 95.8675)
  line L4 (-60, 95.8675) -> (-57.25, 95.8675)
  line L5 (-57.25, 95.8675) -> (0, 95.8675)
  line L6 (-64, 123.2917) -> (-64, 136.282)
  line L7 (-64, 136.282) -> (-64, 152.6218)
  line L8 (-64, 167.6218) -> (-64, 152.6218)
  line L9 (-64, 70.1218) -> (-64, 123.2917)
  line L10 (0, 124.2446) -> (-64, 124.2446) construction
  line L11 (-32, 124.2446) -> (-32, 152.6218) construction
  circle A0 centre (-48, 124.2446) radius 6
  circle A1 centre (-16, 124.2446) radius 6
  circle A2 centre (-48, 124.2446) radius 8 construction
  circle A3 centre (-16, 124.2446) radius 8 construction
  dimension "d228_1" = 12
  dimension "d229_1" = 16
  dimension "d230_1" = 32
  dimension "d233_1" = 16
  constraint midpoint L0 L10.start
  constraint coincident L6 L10.end
  constraint perpendicular L6 L10
  constraint midpoint L10 L11.start
  constraint coincident L1 L11.end
  constraint perpendicular L1 L11
  constraint coincident L10 A0.centre
  constraint symmetric L11 A0 A1
  constraint concentric A0 A2
  constraint symmetric L11 A2 A3
  measures "d228_1" diameter of A0
  measures "d229_1" distance of L9 A0.centre
  measures "d230_1" distance of A0.centre A1.centre
  measures "d233_1" diameter of A2
extrude "Extrude21''" [suppressed] in component "Scanner GM67"
extrude "Extrude22''" [suppressed] in component "Scanner GM67"
fillet "Fillet6''" [suppressed] in component "Scanner GM67"
extrude "Extrude23''" [suppressed] in component "Scanner GM67"
extrude "Extrude20'" [suppressed] in component "Scanner GM67"
component "GM60 standalone" placed x (1, 0, 0) y (0, 1, 0) z (0, 0, 1) at (0, 0, 0)
component "Sample display" placed x (1, 0, 0) y (0, 1, 0) z (0, 0, 1) at (0, 0, 0)
component "LID" placed x (1, 0, 0) y (0, 1, 0) z (0, 0, 1) at (0, 0, 0)
component "GM67" placed x (1, 0, 0) y (0, 1, 0) z (0, 0, 1) at (0, 0, 0)
component "Trial printer" placed x (1, 0, 0) y (0, 1, 0) z (0, 0, 1) at (0, 0, 0)
component "GM67 + printer" placed x (1, 0, 0) y (0, 1, 0) z (0, 0, 1) at (0, 0, 0)
component "Trial scanner" placed x (1, 0, 0) y (0, 1, 0) z (0, 0, 1) at (0, 0, 0)
component "Powersupply" placed x (1, 0, 0) y (0, 1, 0) z (0, 0, 1) at (44.3976, 24.2447, 62.2555)
component "display trial" placed x (1, 0, 0) y (0, 1, 0) z (0, 0, 1) at (0, 0, 0)
component "Bottom LID - Printer" placed x (1, 0, 0) y (0, 1, 0) z (0, 0, 1) at (0, 0, 0)
component "Top lid" placed x (1, 0, 0) y (0, 1, 0) z (0, 0, 1) at (0, 0, 0)
hidden bodies 14 15 20
equation "d3 = d2"
equation "d73 = -( 4 mm - 2 mm )"
equation "d75 = -( 4 mm - 0.6 mm )"
equation "d97 = d94"
equation "d112 = d111"
equation "d115 = d105"
equation "d148 = d147"
equation "d149 = d147"
equation "d150 = d147"
equation "d151 = d147"
equation "d157 = d147"
equation "d3_1 = d2_1"
equation "d73_1 = -( 4 mm - 2 mm )"
equation "d75_1 = -( 4 mm - 0.6 mm )"
equation "d97_1 = d94_1"
equation "d112_1 = d111_1"
equation "d115_1 = d105_1"
equation "d148_1 = d147_1"
equation "d149_1 = d147_1"
equation "d150_1 = d147_1"
equation "d151_1 = d147_1"
equation "d157_1 = d147_1"
equation "d3_2 = d2_2"
equation "d73_2 = -( 4 mm - 2.9 mm )"
equation "d75_2 = -( 4 mm - 1.5 mm )"
equation "d112_2 = d111_2"
equation "d115_2 = d105_2"
equation "d120_2 = d84_3"
equation "d148_2 = d147_2"
equation "d149_2 = d147_2"
equation "d150_2 = d147_2"
equation "d157_2 = d147_2"
equation "d393 = d9_2"
equation "d413 = d412"
equation "d432 = ( 17.1 / 2 ) * 1 mm"
equation "d466 = d85_2"
equation "d467 = d147_2"
equation "d468 = d465"
equation "d469 = d85_2"
equation "d470 = d147_2"
equation "d478 = d84_3"
equation "d479 = d85_2"
equation "d480 = d147_2"
equation "d489 = d85_2"
equation "d490 = d147_2"
equation "d493 = d84_3"
equation "d510 = d84_3"
equation "d512 = d85_2"
equation "d513 = d147_2"
equation "d515 = d84_3"
equation "d516 = d85_2"
equation "d517 = d147_2"
equation "d550 = 16.25 mm - 3 mm"
equation "d563 = d583 / 2"
equation "d624 = d623"
equation "d625 = d623"
equation "d626 = d623"
equation "d634 = d633"
equation "d635 = d633"
equation "d636 = d633"
equation "d648 = d647"
equation "d649 = d647"
equation "d650 = d647"
equation "d659 = d658"
equation "d665 = d633"
equation "d666 = d633"
equation "d667 = d633"
equation "d671 = d633"
equation "d672 = d633"
equation "d673 = d633"
named bodies: "Body1 (1)"
